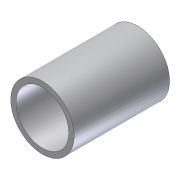
# Autodesk Inventor part: FE-00002-09
Saved by Autodesk Inventor 2012 (Build 160160000, 160)
## iProperties
Created: 2008-05-15
Part Number: FE-00002-09
Document SubType Name: Modeling
Designer: narosenberg
Density: 1 g/cm^3
Mass: 27.3881 g
Surface Area: 162.665 cm^2
Volume: 27.3881 cm^3
Material: Default
Author: narosenberg
Autodesk Inventor part; units mm, degrees
ref_plane "YZ Plane" through (0, 0, 0) normal (1, 0, 0) x (0, 1, 0)
ref_plane "XZ Plane" through (0, 0, 0) normal (0, 1, 0) x (-1, 0, 0)
ref_plane "XY Plane" through (0, 0, 0) normal (0, 0, 1) x (1, 0, 0)
sketch "Sketch1" plane through (0, 0, 0) normal (0, 0, 1) x (1, 0, 0)
  circle A0 centre (-16.129, 5.6068) radius 21.082
  dimension "d0" = 42.164
  constraints: 1 centre point
  measures "d0" diameter of A0
extrude "Extrusion1" add sketch "Sketch1" along normal blind 63.5
shell "Shell1" thickness 3.556 removed faces 2 at (-10.2683, -0.6372, 0) at (-10.2683, -0.6372, 63.5)
body "Solid1"
